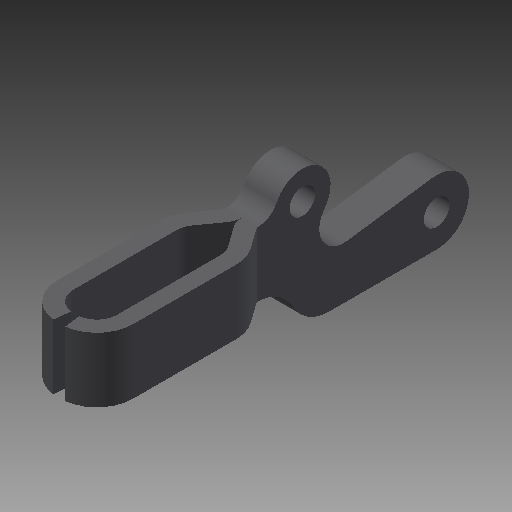
# Autodesk Inventor part: 305106_7-KOMP
Saved by Autodesk Inventor 2018 (Build 220112000, 112)
## iProperties
Category: PARTsolutions
Company: DESTACO
Created: 2018-01-28
Part Number: 305106_7-KOMP
Catalog Web Link: www.cadenas.de
Description: 305106_7-KOMP-U-Spannarm
Vendor: DESTACO
Document SubType Name: Modeling
Designer: psAdmin
Manufacturer: DESTACO
Mass: 1.62907 g
Surface Area: 17.8358 cm^2
Volume: 1.62907 cm^3
Density: 1 g/cm^3
Material: Generic
Appearance: PSOLRGB-192-192-192
PSOL_IDENT_0: {$CADENAS_DATA\23d-libs\destaco\destaco_gmbh\man_spann\horizontalspanner\kompakt\u_kompakt_parts\u_s
PSOL_IDENT_1: pannarm_u_komp.prj},168 {VTYP=3D},{NB=305106_7-KOMP},{LINA=305106_7-KOMP},{NN=305106_7-KOMP},{DATE=2
PSOL_IDENT_2: 0.09.2016 07:53:11},{GEOMDATE=27.06.2006},{VERSION=v1},{LINEID=10},{LINESUBID=-1},{WBVAR=}  {NB=3051
PSOL_IDENT_3: 06_7-KOMP},{LINA=305106_7-KOMP},{KT=DUMMY},{MODELL=305106_7-KOMP},{SIZE=1.000}
NN: 305106_7-KOMP
NT: U-Spannarm
NB: 305106_7-KOMP
NBSYN: $MODELL.
LINA: 305106_7-KOMP
MODELL: 305106_7-KOMP
SIZE: 1.000
SUPPLIER: DESTACO
ARTICLENO: 305106_7-KOMP
BOMINFO: 305106_7-KOMP
CREATOR: CADENAS GmbH
Title: 305106_7-KOMP
Author: Cadenas PARTsolutions
Comments: U-Spannarm
Autodesk Inventor part; units mm, degrees
sketch "Skizze_1" plane through (0, 0, 0) normal (0, 1, 0) x (-1, 0, 0)
  line L0 (4.7, 27.5428) -> (4.7, 40.3427)
  arc A0 (4.7, 40.3427) -> (0.7437, 44.8097) centre (0.2, 40.3427) ccw
  line L1 (0.7437, 44.8097) -> (0.5, 42.8246)
  arc A1 (2.7, 40.3427) -> (0.5, 42.8246) centre (0.2, 40.3427) ccw
  line L2 (2.7, 40.3427) -> (2.7, 27.5428)
  arc A2 (2.2372, 26.0938) -> (2.7, 27.5428) centre (0.2, 27.5428) ccw
  line L3 (2.2372, 26.0938) -> (0.4628, 23.599)
  arc A3 (0.4628, 23.599) -> (0, 22.15) centre (2.5, 22.15) ccw
  arc A4 (0, 22.15) -> (-0.4628, 23.599) centre (-2.5, 22.15) ccw
  line L4 (-0.4628, 23.599) -> (-2.2372, 26.0938)
  arc A5 (-2.7, 27.5428) -> (-2.2372, 26.0938) centre (-0.2, 27.5428) ccw
  line L5 (-2.7, 27.5428) -> (-2.7, 40.3427)
  arc A6 (-0.5, 42.8246) -> (-2.7, 40.3427) centre (-0.2, 40.3427) ccw
  line L6 (-0.5, 42.8246) -> (-0.7437, 44.8097)
  arc A7 (-0.7437, 44.8097) -> (-4.7, 40.3427) centre (-0.2, 40.3427) ccw
  line L7 (-4.7, 40.3427) -> (-4.7, 27.5428)
  arc A8 (-4.7, 27.5428) -> (-3.867, 24.9345) centre (-0.2, 27.5428) ccw
  line L8 (-3.867, 24.9345) -> (-2.0926, 22.4398)
  arc A9 (-2, 22.15) -> (-2.0926, 22.4398) centre (-2.5, 22.15) ccw
  line L9 (-2, 22.15) -> (-2, -4)
  line L10 (-2, -4) -> (2, -4)
  line L11 (2, -4) -> (2, 22.15)
  arc A10 (2.0926, 22.4398) -> (2, 22.15) centre (2.5, 22.15) ccw
  line L12 (2.0926, 22.4398) -> (3.867, 24.9345)
  arc A11 (3.867, 24.9345) -> (4.7, 27.5428) centre (0.2, 27.5428) ccw
  constraints: 26 end point, 24 point on circle, 12 centre point
extrude "Extrusion1" add sketch "Skizze_1" along normal mid plane 40
sketch "Skizze_2" plane through (0, 0, 0) normal (1, 0, 0) x (0, 1, 0)
  line L0 (-60, 105) -> (-60, -73)
  line L1 (-60, -73) -> (65, -73)
  line L2 (65, -73) -> (65, 105)
  line L3 (65, 105) -> (-60, 105)
  line L4 (1.5, 44.8175) -> (1.5, 22.25)
  arc A0 (-1.25, 17.7848) -> (1.5, 22.25) centre (-3.5, 22.25) ccw
  arc A1 (-1.25, 17.7848) -> (-4, 13.3197) centre (1, 13.3197) ccw
  line L5 (-4, 13.3197) -> (-4, 0)
  arc A2 (-4, 0) -> (3.9611, 0.5567) centre (0, 0) ccw
  line L6 (3.9611, 0.5567) -> (2.4717, 11.1545)
  arc A3 (7.3248, 13.908) -> (2.4717, 11.1545) centre (5.4425, 11.572) ccw
  arc A4 (7.3248, 13.908) -> (10.9583, 19.8317) centre (9.5, 16.65) ccw
  arc A5 (9.5, 22.1044) -> (10.9583, 19.8317) centre (12, 22.1044) ccw
  line L7 (9.5, 22.1044) -> (9.5, 44.8175)
  line L8 (9.5, 44.8175) -> (1.5, 44.8175)
  constraints: 18 end point, 12 point on circle, 6 centre point
extrude "Extrusion2" cut sketch "Skizze_2" along normal mid plane 40
sketch "Skizze_3_ALT_Drilling_1" plane through (0, 0, 0) normal (0, 1, 0) x (-1, 0, 0)
  line L0 (-10, 0) -> (10, 0)
  line L1 (10, 0) -> (10, -1.6)
  line L2 (10, -1.6) -> (-10, -1.6)
  line L3 (-10, -1.6) -> (-10, 0)
  line L4 (-10, 0) -> (10, 0)
  constraints: 10 end point
revolve "Revolution1" cut sketch "Skizze_3_ALT_Drilling_1" angle 360 about axis through (10, 0, 0) along (1, 0, 0)
sketch "Skizze_4_ALT_Drilling_2" plane through (0, 0, 16.65) normal (0, 0, 1) x (1, 0, 0)
  line L0 (10, 9.5) -> (-10, 9.5)
  line L1 (-10, 9.5) -> (-10, 11.1)
  line L2 (-10, 11.1) -> (10, 11.1)
  line L3 (10, 11.1) -> (10, 9.5)
  line L4 (10, 9.5) -> (-10, 9.5)
  constraints: 10 end point
revolve "Revolution2" cut sketch "Skizze_4_ALT_Drilling_2" angle 360 about axis through (10, 9.5, 16.65) along (1, 0, 0)
ref_plane "P1_XY" through (0, 9.5, 34.5093) normal (0, 1, 0) x (1, 0, 0)
ref_plane "P1_YZ" through (0, 9.5, 34.5093) normal (1, 0, 0) x (0, 0, -1)
ref_plane "P1_ZX" through (0, 9.5, 34.5093) normal (0, 0, -1) x (0, 1, 0)
ref_plane "P2_XY" through (0, 1.5, 34.5093) normal (0, 1, 0) x (1, 0, 0)
ref_plane "P2_YZ" through (0, 1.5, 34.5093) normal (1, 0, 0) x (0, 0, -1)
ref_plane "P2_ZX" through (0, 1.5, 34.5093) normal (0, 0, -1) x (0, 1, 0)
ref_plane "SA1_XY" through (0, 0, 0) normal (1, 0, 0) x (0, 0, -1)
ref_plane "SA1_YZ" through (0, 0, 0) normal (0, 0, -1) x (0, 1, 0)
ref_plane "SA1_ZX" through (0, 0, 0) normal (0, 1, 0) x (1, 0, 0)
ref_plane "SA2_XY" through (0, 9.5, 16.65) normal (1, 0, 0) x (0, 0, -1)
ref_plane "SA2_YZ" through (0, 9.5, 16.65) normal (0, 0, -1) x (0, 1, 0)
ref_plane "SA2_ZX" through (0, 9.5, 16.65) normal (0, 1, 0) x (1, 0, 0)
ref_plane "SA3_XY" through (0, 5.5, 34.5093) normal (0, 0, 1) x (1, 0, 0)
ref_plane "SA3_YZ" through (0, 5.5, 34.5093) normal (1, 0, 0) x (0, 1, 0)
ref_plane "SA3_ZX" through (0, 5.5, 34.5093) normal (0, 1, 0) x (0, 0, 1)
body "Solid1"
